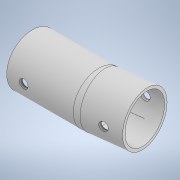
# Autodesk Inventor part: airfoil
Saved by Autodesk Inventor 2022 (Build 260153000, 153)
## iProperties
Created: 2021-03-06
Part Number: airfoil
Material: Generic
Document SubType Name: Modeling
Designer: Ferdinand Hubbard
Density: 1 g/cm^3
Appearance: Default
Author: Ferdinand Hubbard
Autodesk Inventor part; units mm, degrees
ref_plane "YZ Plane" through (0, 0, 0) normal (1, 0, 0) x (0, 1, 0)
ref_plane "XZ Plane" through (0, 0, 0) normal (0, 1, 0) x (-1, 0, 0)
ref_plane "XY Plane" through (0, 0, 0) normal (0, 0, 1) x (1, 0, 0)
sketch "Sketch5" plane through (0, 0, 0) normal (0, 1, 0) x (-1, 0, 0)
  line L0 (0, 0) -> (-23.3884, 0)
  line L1 (-24.6071, -0.0745) -> (-37.8956, -1.7062)
  arc A0 (-23.3884, 0) -> (-24.6071, -0.0745) centre (-23.3884, -10) ccw
  point P0 (-24, 0)
  dimension "d122" = 24
  dimension "d123" = 14
  dimension "d124" = 173
  dimension "d125" = 10
  constraints: 4 end point, 2 point on circle, 2 point on line, 2 tangent, 1 centre point, 1 horizontal
  measures "d122" distance of L0.start point (-24, 0)
  measures "d123" distance of point (-24, 0) L1.end
  measures "d124" angle of L1 L0
  measures "d125" radius of A0
sketch "Sketch6" plane through (0, 0, 0) normal (1, 0, 0) x (0, 1, 0)
  circle A0 centre (0, 0) radius 8
  circle A1 centre (0, 0) radius 9
  line L0 (-0.005, -0.005) -> (0.005, -0.005)
  line L1 (0.005, -0.005) -> (0.005, 0.005)
  line L2 (0.005, 0.005) -> (-0.005, 0.005)
  line L3 (-0.005, 0.005) -> (-0.005, -0.005)
  line L4 (-0.005, -0.005) -> (0.005, 0.005) construction
  line L5 (0.005, -0.005) -> (-0.005, 0.005) construction
  dimension "d126" = 16
  dimension "d127" = 18
  dimension "d138" = 0.01
  dimension "d139" = 0.01
  constraints: 12 end point, 2 centre point, 2 coincident, 2 midpoint, 2 parallel, 1 horizontal, 1 perpendicular
  measures "d126" diameter of A0
  measures "d127" diameter of A1
  measures "d138" distance of L2.end L0.start
  measures "d139" distance of L0.start L0.end
sweep "Sweep1" add profiles "Sketch6" path "Sketch5" path curves L0 A0 L1
sketch "Sketch7" plane through (0, 0, 0) normal (0, 0, 1) x (1, 0, 0)
  line L0 (0, 0) -> (6, 0) construction
  circle A0 centre (6, 0) radius 1.5
  dimension "d130" = 6
  dimension "d131" = 3
  constraints: 2 end point, 1 centre point, 1 coincident, 1 horizontal
  measures "d130" distance of L0.start L0.end
  measures "d131" diameter of A0
extrude "Extrusion8" cut sketch "Sketch7" along normal mid plane 25
sketch "Sketch8" plane through (24.6065, -0.005, -0.0795) normal (-0.1218693, 0, -0.9925462) x (-0.9925462, 0, 0.1218693)
  line L0 (-13.3884, 0) -> (-13.3884, 0.01) projected
  line L1 (-13.3884, 0.005) -> (-7.3884, 0.005) construction
  circle A0 centre (-7.3884, 0.005) radius 1.5
  point P0 (24.4327, 0.005)
  dimension "d134" = 6
  dimension "d135" = 3
  constraints: 2 end point, 1 centre point, 1 coincident, 1 horizontal, 1 midpoint
  measures "d134" distance of L1.start L1.end
  measures "d135" diameter of A0
extrude "Extrusion9" cut sketch "Sketch8" along normal mid plane 25
body "Solid7"
